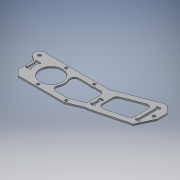
# Autodesk Inventor part: 足首_メインフレーム_1_1
Saved by Autodesk Inventor 2018 (Build 220112000, 112)
## iProperties
Created: 2016-04-30
Part Number: 足首_メインフレーム_1_1
Material: アルミニウム 2014-T4
Document SubType Name: Modeling
Designer: hiroaki
Density: 2.8 g/cm^3
Appearance: サテン
Mass: 6.61842 g
Surface Area: 42.008 cm^2
Volume: 2.36372 cm^3
d0: 1.000 ul
d1: 3.100 mm
d2: 3.000 mm
d3: 11.000 mm
d4: 0.025 mm
d5: 2.100 mm
d6: 21.500 mm
d7: 2.000 mm
d9: 10.000 mm
d11: 10.000 mm
d14: 0.025 mm
d15: 2.100 mm
d18: 22.000 mm
d20: 2.000 mm
d21: 0.025 mm
d22: 5.600 mm
d23: 1.000 mm
d25: 1.000 mm
d27: 5.000 mm
d28: 5.000 mm
d29: 2.000 mm
d30: 5.000 mm
d31: 5.000 mm
d32: 135.00 deg
d33: 1.500 mm
d34: 0.00 deg
d35: 6.100 mm
d36: 2.100 mm
d37: 6.000 ul
d39: 360.00 deg
d41: 0.250 mm
d42: 0.00 deg
d43: 3.500 mm
Author: hiroaki
Autodesk Inventor part; units mm, degrees
ref_plane "YZ Plane" through (0, 0, 0) normal (1, 0, 0) x (0, 1, 0)
ref_plane "XZ Plane" through (0, 0, 0) normal (0, 1, 0) x (-1, 0, 0)
ref_plane "XY Plane" through (0, 0, 0) normal (0, 0, 1) x (1, 0, 0)
derived "下半身全体像_1_1.ipt"
sketch "スケッチ1" plane through (0, 0, 0) normal (0, 0, 1) x (1, 0, 0)
  circle A0 centre (0, 0) radius 10.5 construction
  line L0 (0, 0) -> (-12, 0) construction
  arc A1 (0, 16) -> (-12, 10.583) centre (0, 0) ccw construction
  arc A2 (-12, -10.583) -> (0, -16) centre (0, 0) ccw construction
  line L1 (0, 16) -> (39.5, 16) construction
  line L2 (39.5, 16) -> (39.5, -16) construction
  line L3 (39.5, -16) -> (0, -16) construction
  circle A3 centre (1, 13.5) radius 1.35 projected
  circle A4 centre (1, -13.5) radius 1.35 projected
  circle A5 centre (28, 13.5) radius 1.35 projected
  circle A6 centre (28, -13.5) radius 1.35 projected
  line L4 (1, 13.5) -> (1, -13.5) construction
  line L5 (1, -13.5) -> (28, -13.5) construction
  line L6 (1, 13.5) -> (28, 13.5) construction
  line L7 (28, 13.5) -> (28, -13.5) construction
  line L8 (0, 0) -> (1, 0) construction
  line L9 (32, 120) -> (32, 20) construction
  line L10 (0, 0) -> (0, 0) construction
  circle A7 centre (32, 120) radius 4.05 projected
  line L11 (0, 140) -> (0, 40) construction
  circle A8 centre (0, 40) radius 4.05 projected
  line L12 (0, 0) -> (0, -100) construction
  line L13 (32, 20) -> (32, -80) construction
  line L14 (0, 0) -> (0, 40) construction
  circle A9 centre (32, 20) radius 6.5 construction
  line L15 (32, 23.5218) -> (35.05, 21.7609) construction
  line L16 (35.05, 21.7609) -> (35.05, 18.2391) construction
  line L17 (35.05, 18.2391) -> (32, 16.4782) construction
  line L18 (32, 16.4782) -> (28.95, 18.2391) construction
  line L19 (28.95, 18.2391) -> (28.95, 21.7609) construction
  line L20 (28.95, 21.7609) -> (32, 23.5218) construction
  line L21 (21.5, 152) -> (61, 152) construction
  line L22 (61, 152) -> (61, 100.5) construction
  line L23 (61, 100.5) -> (21.5, 100.5) construction
  line L24 (21.5, 100.5) -> (21.5, 152) construction
  line L25 (21.5, 140) -> (61, 140) construction
  line L26 (16, 150.5) -> (66.5, 150.5) construction
  line L27 (66.5, 150.5) -> (66.5, 129.5) construction
  line L28 (66.5, 129.5) -> (16, 129.5) construction
  line L29 (16, 129.5) -> (16, 150.5) construction
  circle A10 centre (0, 140) radius 10.5 construction
  line L30 (-13.5, 139) -> (13.5, 139) construction
  line L31 (13.5, 139) -> (13.5, 112) construction
  line L32 (13.5, 112) -> (-13.5, 112) construction
  line L33 (-13.5, 112) -> (-13.5, 139) construction
  circle A11 centre (-13.5, 139) radius 1.35 projected
  circle A12 centre (13.5, 139) radius 1.35 projected
  circle A13 centre (-13.5, 112) radius 1.35 projected
  circle A14 centre (13.5, 112) radius 1.35 projected
  line L34 (-12, 10.583) -> (-12, -10.583) construction
  circle A15 centre (0, -100) radius 4.05 construction
  circle A16 centre (32, -80) radius 4.05 construction
  circle A17 centre (0, -100) radius 10.5 construction
  line L35 (32, -80) -> (0, -100) construction
  line L36 (45, -60.5) -> (77.5, -60.5) construction
  line L37 (77.5, -60.5) -> (77.5, -112) construction
  line L38 (77.5, -112) -> (45, -112) construction
  line L39 (45, -112) -> (45, -60.5) construction
  line L40 (45, -100) -> (77.5, -100) construction
  line L41 (39.5, -89.5) -> (83, -89.5) construction
  line L42 (83, -89.5) -> (83, -110.5) construction
  line L43 (83, -110.5) -> (39.5, -110.5) construction
  line L44 (39.5, -110.5) -> (39.5, -89.5) construction
  line L45 (1, -86.5) -> (28, -86.5) construction
  line L46 (28, -86.5) -> (28, -113.5) construction
  line L47 (28, -113.5) -> (1, -113.5) construction
  line L48 (1, -113.5) -> (1, -86.5) construction
  circle A18 centre (1, -86.5) radius 1.35 projected
  circle A19 centre (1, -113.5) radius 1.35 projected
  circle A20 centre (28, -113.5) radius 1.35 projected
  circle A21 centre (28, -86.5) radius 1.35 projected
  circle A22 centre (32, 20) radius 4.05 projected
  circle A23 centre (32, 20) radius 4.05 projected
  line L49 (10.583, 152) -> (-10.583, 152) construction
  line L50 (16, 140) -> (16, 100.5) construction
  line L51 (16, 100.5) -> (-16, 100.5) construction
  line L52 (-16, 100.5) -> (-16, 140) construction
  arc A24 (16, 140) -> (10.583, 152) centre (0, 140) ccw construction
  arc A25 (-10.583, 152) -> (-16, 140) centre (0, 140) ccw construction
  line L53 (-12, -89.417) -> (-12, -110.583) construction
  line L54 (0, -84) -> (39.5, -84) construction
  line L55 (39.5, -84) -> (39.5, -116) construction
  line L56 (39.5, -116) -> (0, -116) construction
  arc A26 (0, -84) -> (-12, -89.417) centre (0, -100) ccw construction
  arc A27 (-12, -110.583) -> (0, -116) centre (0, -100) ccw construction
  circle A28 centre (-8.5, 0) radius 1.35 projected
  circle A29 centre (0, 0) radius 8.5 construction
  line L57 (35.05, 121.7609) -> (35.05, 118.2391) construction
  line L58 (35.05, 118.2391) -> (32, 116.4782) construction
  line L59 (32, 116.4782) -> (28.95, 118.2391) construction
  line L60 (28.95, 118.2391) -> (28.95, 121.7609) construction
  line L61 (28.95, 121.7609) -> (32, 123.5218) construction
  line L62 (32, 123.5218) -> (35.05, 121.7609) construction
  line L63 (0, 152) -> (0, 140) construction
  line L64 (0, 140) -> (0, 139) construction
  circle A30 centre (83.3, -84.5) radius 1.55
  line L65 (-19, -94.5) -> (-16, -94.5) construction
  line L66 (-16, -94.5) -> (-16, -105.5) construction
  line L67 (-16, -105.5) -> (-19, -105.5) construction
  line L68 (-19, -105.5) -> (-19, -94.5) construction
  line L69 (-15.975, -94.475) -> (-19.025, -94.475) construction
  line L70 (-19.025, -94.475) -> (-19.025, -105.525) construction
  line L71 (-19.025, -105.525) -> (-15.975, -105.525) construction
  line L72 (-15.975, -105.525) -> (-15.975, -94.475) construction
  circle A31 centre (-19.025, -95.525) radius 1.05 construction
  arc A32 (-19.025, -94.475) -> (-19.025, -96.575) centre (-19.025, -95.525) ccw
  line L73 (-19.025, -94.475) -> (-15.975, -94.475)
  arc A33 (-15.975, -96.575) -> (-15.975, -94.475) centre (-15.975, -95.525) ccw
  line L74 (-17.5, -94.475) -> (-17.5, -105.525) construction
  line L75 (-15.975, -96.575) -> (-15.975, -103.425)
  line L76 (-19.025, -96.575) -> (-19.025, -103.425)
  arc A34 (-19.025, -103.425) -> (-19.025, -105.525) centre (-19.025, -104.475) ccw
  arc A35 (-15.975, -105.525) -> (-15.975, -103.425) centre (-15.975, -104.475) ccw
  line L77 (-19.025, -105.525) -> (-15.975, -105.525)
  circle A36 centre (0, -100) radius 10.75
  line L78 (43, -95) -> (45, -95) construction
  line L79 (45, -95) -> (45, -105) construction
  line L80 (45, -105) -> (43, -105) construction
  line L81 (43, -105) -> (43, -95) construction
  line L82 (45, -95) -> (39.5, -95) construction
  line L83 (39.5, -95) -> (39.5, -105) construction
  line L84 (39.5, -105) -> (45, -105) construction
  line L85 (45, -105) -> (45, -95) construction
  line L86 (45.025, -94.975) -> (42.975, -94.975) construction
  line L87 (42.975, -94.975) -> (42.975, -105.025) construction
  line L88 (42.975, -105.025) -> (45.025, -105.025) construction
  line L89 (45.025, -105.025) -> (45.025, -94.975) construction
  circle A37 centre (42.975, -96.025) radius 1.05 construction
  line L90 (42.975, -94.975) -> (45.025, -94.975)
  arc A38 (42.975, -94.975) -> (42.975, -97.075) centre (42.975, -96.025) ccw
  arc A39 (45.025, -97.075) -> (45.025, -94.975) centre (45.025, -96.025) ccw
  line L91 (44, -95) -> (44, -105.025) construction
  line L92 (42.975, -97.075) -> (42.975, -102.925)
  line L93 (45.025, -97.075) -> (45.025, -102.925)
  line L94 (42.975, -105.025) -> (45.025, -105.025)
  arc A40 (42.975, -102.925) -> (42.975, -105.025) centre (42.975, -103.975) ccw
  arc A41 (45.025, -105.025) -> (45.025, -102.925) centre (45.025, -103.975) ccw
  line L95 (77.5, -96.5) -> (45, -96.5) construction
  line L96 (77.5, -74.5) -> (79.5, -74.5) construction
  line L97 (79.5, -74.5) -> (79.5, -96.5) construction
  line L98 (79.5, -96.5) -> (77.5, -96.5) construction
  line L99 (77.5, -96.5) -> (77.5, -74.5) construction
  line L100 (45, -74.5) -> (77.5, -74.5) construction
  line L101 (79.525, -74.475) -> (77.475, -74.475) construction
  line L102 (77.475, -74.475) -> (77.475, -96.525) construction
  line L103 (77.475, -96.525) -> (79.525, -96.525) construction
  line L104 (79.525, -96.525) -> (79.525, -74.475) construction
  circle A42 centre (77.475, -75.525) radius 1.05 construction
  line L105 (77.475, -74.475) -> (79.525, -74.475)
  arc A43 (77.475, -74.475) -> (77.475, -76.575) centre (77.475, -75.525) ccw
  line L106 (77.475, -76.575) -> (77.475, -94.425)
  arc A44 (79.525, -76.575) -> (79.525, -74.475) centre (79.525, -75.525) ccw
  line L107 (79.525, -76.575) -> (79.525, -94.425)
  line L108 (78.5, -74.475) -> (78.5, -89.5) construction
  line L109 (79.525, -85.5) -> (77.475, -85.5) construction
  arc A45 (77.475, -94.425) -> (77.475, -96.525) centre (77.475, -95.475) ccw
  line L110 (77.475, -96.525) -> (79.525, -96.525)
  arc A46 (79.525, -96.525) -> (79.525, -94.425) centre (79.525, -95.475) ccw
  line L111 (83.3, -81.2668) -> (86.1, -82.8834) construction
  line L112 (86.1, -82.8834) -> (86.1, -86.1166) construction
  line L113 (86.1, -86.1166) -> (83.3, -87.7332) construction
  line L114 (83.3, -87.7332) -> (80.5, -86.1166) construction
  line L115 (80.5, -86.1166) -> (80.5, -82.8834) construction
  line L116 (80.5, -82.8834) -> (83.3, -81.2668) construction
  line L117 (-21, -95.2931) -> (-21, -110.5)
  line L118 (-21, -110.5) -> (-16, -116)
  line L119 (-16, -116) -> (28.4967, -116)
  line L120 (28.4967, -116) -> (43, -110)
  line L121 (43, -110) -> (45, -110)
  line L122 (87.1, -85.3494) -> (87.1, -75.6858)
  line L123 (76.7437, -69.5) -> (39.5, -84)
  line L124 (39.5, -84) -> (-16, -84)
  circle A47 centre (1, -86.5) radius 2.5 construction
  circle A48 centre (28, -113.5) radius 2.5 construction
  circle A49 centre (43, -110) radius 2 construction
  circle A50 centre (79.5, -101.5) radius 1 construction
  line L125 (80.9142, -69.5) -> (87.1, -75.6858)
  circle A51 centre (79.5, -69.5) radius 1 construction
  line L126 (76.7437, -69.5) -> (80.9142, -69.5)
  line L127 (45, -110) -> (77.5, -101.5)
  line L128 (77.5, -101.5) -> (79.5, -101.5)
  line L129 (79.5, -101.5) -> (87.1, -85.3494)
  circle A52 centre (83.3, -84.5) radius 3.8 construction
  line L130 (0, -100) -> (1, -100) construction
  line L131 (-19.5, -90.6166) -> (-22.3, -92.2332)
  line L132 (-22.3, -92.2332) -> (-25.1, -90.6166)
  line L133 (-25.1, -90.6166) -> (-25.1, -87.3834)
  line L134 (-25.1, -87.3834) -> (-22.3, -85.7668)
  line L135 (-22.3, -85.7668) -> (-19.5, -87.3834)
  line L136 (-19.5, -87.3834) -> (-19.5, -90.6166)
  circle A53 centre (-22.3, -89) radius 1.55
  line L137 (-21, -95.2931) -> (-27.1, -91.7713)
  line L138 (-27.1, -91.7713) -> (-27.1, -86.2287)
  line L139 (-27.1, -86.2287) -> (-23.2397, -84)
  line L140 (-23.2397, -84) -> (-16, -84)
  point P0 (66.5, 140)
  point P1 (39.5, 0)
  point P2 (83, -100)
  point P3 (-12, -100)
  point P4 (39.5, -100)
  point P5 (-19, -100)
  point P6 (39.5, -100)
  point P7 (78.5, -85.5)
  point P8 (-19.025, -100)
  dimension "d5" = 2.1
  dimension "d15" = 2.1
  dimension "d1" = 3.1
  dimension "d2" = 3
  dimension "d3" = 11
  dimension "d4" = 0.025
  dimension "d6" = 21.5
  dimension "d7" = 2
  dimension "d9" = 10
  dimension "d11" = 10
  dimension "d14" = 0.025
  dimension "d18" = 22
  dimension "d20" = 2
  dimension "d21" = 0.025
  dimension "d22" = 5.6
  dimension "d23" = 1
  dimension "d25" = 1
  dimension "d28" = 5
  dimension "d29" = 2
  dimension "d30" = 5
  dimension "d31" = 5
  dimension "d32" = 135
  dimension "d43" = 3.5
  dimension "d58" = 2
  dimension "d59" = 5
  dimension "d60" = 5.6
  dimension "d61" = 3.1
  dimension "d64" = 0.5
  dimension "d65" = 2
  dimension "d66" = 2
  dimension "d67" = 5.5
  dimension "d68" = 2
  dimension "d76" = 1
  dimension "d77" = 4
  constraints: 152 end point, 24 point on circle, 21 centre point, 18 parallel, 15 horizontal, 15 point on line, 14 perpendicular, 13 collinear, 12 midpoint, 11 tangent, 10 vertical, 10 vertical alignment, 9 coincident, 9 symmetric about line, 7 equal radius, 2 horizontal alignment, 53 other
  measures "d1" diameter of A30
  measures "d2" distance of L65.start L65.end
  measures "d3" distance of L67.end L65.start
  measures "d4" distance between parallel lines of L69 L65
  measures "d6" diameter of A36
  measures "d7" distance of L78.start L78.end
  measures "d9" distance of L82.end L83.end
  measures "d11" distance of L80.end L78.start
  measures "d14" distance between parallel lines of L86 L78
  measures "d18" distance between parallel lines of L100 L95
  measures "d20" distance of L96.start L96.end
  measures "d21" distance between parallel lines of L101 L96
  measures "d22" distance between parallel lines of L115 L112
  measures "d23" distance between parallel lines of L115 L97
  measures "d25" distance between parallel lines of L122 L112
  measures "d28" distance of L80.end A49.centre
  measures "d29" diameter of A50
  measures "d30" distance of L97.end A50.centre
  measures "d31" distance of L96.end A51.centre
  measures "d32" angle of L122 L125
  measures "d43" distance between parallel lines of L95 L40
  measures "d58" distance between parallel lines of L68 L117
  measures "d59" distance from line of L117.end L67
  measures "d60" distance between parallel lines of L135 L132
  measures "d61" diameter of A53
  measures "d64" distance between parallel lines of L136 L68
  measures "d65" distance between parallel lines of L137 L132
  measures "d66" distance between parallel lines of L133 L138
  measures "d67" distance from line of L65 point (-22.3, -89)
  measures "d68" distance between parallel lines of L134 L139
  measures "d76" distance from line of L109 A30.centre
  measures "d77" distance between parallel lines of L53 L66
extrude "押し出し1" add sketch "スケッチ1" along normal blind 1.5 contours L137 L138 L139 L140 L124 L123 L126 L125 L122 L129 L128 L127 L121 L120 L119 L118 L117 | L131 L132 L133 L134 L135 L136
sketch "スケッチ3" plane through (39.5, -84, 0) normal (0, 0, -1) x (-1, 0, 0)
  circle A0 centre (-43.8, -0.5) radius 1.55 projected
  line L0 (-40.75, 1.2609) -> (-40.75, -2.2609)
  line L1 (-40.75, -2.2609) -> (-43.8, -4.0218)
  line L2 (-43.8, -4.0218) -> (-46.85, -2.2609)
  line L3 (-46.85, -2.2609) -> (-46.85, 1.2609)
  line L4 (-46.85, 1.2609) -> (-43.8, 3.0218)
  line L5 (-43.8, 3.0218) -> (-40.75, 1.2609)
  circle A1 centre (-43.8, 1.9718) radius 1.05
  circle A2 centre (-45.9407, 0.7359) radius 1.05
  circle A3 centre (-45.9407, -1.7359) radius 1.05
  circle A4 centre (-43.8, -2.9718) radius 1.05
  circle A5 centre (-41.6593, -1.7359) radius 1.05
  circle A6 centre (-41.6593, 0.7359) radius 1.05
  circle A7 centre (61.8, -5) radius 1.55 projected
  line L6 (64.6, -6.6166) -> (61.8, -8.2332)
  line L7 (61.8, -8.2332) -> (59, -6.6166)
  line L8 (59, -6.6166) -> (59, -3.3834)
  line L9 (59, -3.3834) -> (61.8, -1.7668)
  line L10 (61.8, -1.7668) -> (64.6, -3.3834)
  line L11 (64.6, -3.3834) -> (64.6, -6.6166)
  circle A8 centre (61.8, -2.8168) radius 1.05
  circle A9 centre (59.9093, -3.9084) radius 1.05
  circle A10 centre (59.9093, -6.0916) radius 1.05
  circle A11 centre (61.8, -7.1832) radius 1.05
  circle A12 centre (63.6907, -6.0916) radius 1.05
  circle A13 centre (63.6907, -3.9084) radius 1.05
  point P0 (39.5, 84)
  point P1 (-43.8, -0.5)
  point P2 (-46.85, 1.2609)
  point P3 (-46.85, -2.2609)
  point P4 (-43.8, -4.0218)
  point P5 (-40.75, -2.2609)
  point P6 (-40.75, 1.2609)
  point P7 (59, -3.3834)
  point P8 (59, -6.6166)
  point P9 (61.8, -8.2332)
  point P10 (64.6, -6.6166)
  point P11 (64.6, -3.3834)
  dimension "d36" = 2.1
  dimension "d69" = 2.1
  dimension "d35" = 6.1
  dimension "d39" = 360
  dimension "d72" = 360
  dimension "d74" = 5.6
  constraints: 24 end point, 6 vertical alignment, 2 coincident, 2 vertical, 96 other
  measures "d35" distance between parallel lines of L3 L0
  measures "d74" distance between parallel lines of L11 L8
extrude "押し出し2" cut sketch "スケッチ3" against normal blind 0.25 contours A0 A6 L0 A5 | A6 A0 | A0 A6 L5 L0 | A5 L0 L1 A0 | A0 A5 | A0 A1 L5 A6 | L0 A6 | A5 L1 A4 A0 | A5 L0 | A1 A0 | A0 A1 L4 L5 | A6 L5 | A4 L1 L2 A0 | A0 A4 | L1 A5 | A0 A2 L4 A1 | L5 A1 | A4 L2 A3 A0 | A4 L1 | A2 A0 | A0 A2 L3 L4 | A1 L4 | A3 L2 L3 A0 | A0 A3 | L2 A4 | A0 A3 L3 A2 | L4 A2 | A3 L2 | A2 L3 | L3 A3 | A7 A13 L11 A12 | A13 A7 | A7 A13 L10 L11 | A12 L11 L6 A7 | A7 A12 | A7 A8 L10 A13 | L11 A13 | A12 L6 A11 A7 | A12 L11 | A8 A7 | A7 A8 L9 L10 | A13 L10 | A11 L6 L7 A7 | A7 A11 | L6 A12 | A7 A9 L9 A8 | L10 A8 | A11 L7 A10 A7 | A11 L6 | A9 A7 | A7 A9 L8 L9 | A8 L9 | A10 L7 L8 A7 | A7 A10 | L7 A11 | A7 A10 L8 A9 | L9 A9 | A10 L7 | A9 L8 | L8 A10
sketch "スケッチ4" plane through (-23.2397, -84, 1.5) normal (0, 0, 1) x (1, 0, 0)
  circle A0 centre (23.2397, -16) radius 10.75 projected
  line L0 (102.7647, -12.525) -> (100.7147, -12.525) projected
  line L1 (100.7147, 9.525) -> (102.7647, 9.525) projected
  line L2 (68.2647, -21.025) -> (66.2147, -21.025) projected
  line L3 (66.2147, -18.925) -> (66.2147, -13.075) projected
  line L4 (66.2147, -10.975) -> (68.2647, -10.975) projected
  circle A1 centre (51.2397, -2.5) radius 1.35 projected
  circle A2 centre (51.2397, -29.5) radius 1.35 projected
  line L5 (62.7397, 0) -> (0, 0) projected
  line L6 (51.7365, -32) -> (66.2397, -26) projected
  line L7 (68.2397, -26) -> (100.7397, -17.5) projected
  line L8 (99.9834, 14.5) -> (62.7397, 0) projected
  line L9 (29.6866, -5) -> (49.5814, -5)
  arc A3 (49.5814, -5) -> (52.8981, -5) centre (51.2397, -2.5) ccw
  arc A4 (29.6866, -27) -> (29.6866, -5) centre (23.2397, -16) ccw
  line L10 (52.8981, -5) -> (63.2397, -5)
  line L11 (63.2397, -5) -> (63.2397, -21.8301)
  line L12 (63.2397, -21.8301) -> (51.8164, -26.5559)
  arc A5 (51.8164, -26.5559) -> (49.5814, -27) centre (51.2397, -29.5) ccw
  line L13 (29.6866, -27) -> (29.6866, -27)
  line L14 (29.6866, -27) -> (49.5814, -27)
  line L15 (23.2397, -16) -> (66.2147, -16) construction
  line L16 (67.2397, -10.975) -> (67.2397, -21.025) construction
  line L17 (71.2397, -2.0563) -> (71.2397, -20.0472)
  line L18 (71.2397, -20.0472) -> (97.7397, -13.1164)
  line L19 (97.7397, -13.1164) -> (97.7397, 8.2609)
  line L20 (97.7397, 8.2609) -> (71.2397, -2.0563)
  line L21 (101.7397, 9.525) -> (101.7397, -12.525) construction
  point P0 (23.2397, 84)
  dimension "d44" = 5
  dimension "d46" = 2
  dimension "d48" = 3
  dimension "d49" = 4
  dimension "d50" = 5
  dimension "d51" = 4
  dimension "d52" = 4
  dimension "d53" = 5
  dimension "d54" = 5
  constraints: 26 end point, 6 point on circle, 5 midpoint, 4 parallel, 3 centre point, 3 coincident, 2 horizontal, 2 perpendicular, 2 vertical, 1 equal radius, 1 horizontal alignment, 1 symmetric about line, 1 vertical alignment
  measures "d44" distance between parallel lines of L5 L9
  measures "d46" radial gap between concentric circles of A4 A0
  measures "d48" radius of A3
  measures "d49" distance between parallel lines of L16 L11
  measures "d50" distance between parallel lines of L6 L12
  measures "d51" distance between parallel lines of L16 L17
  measures "d52" distance between parallel lines of L21 L19
  measures "d53" distance between parallel lines of L8 L20
  measures "d54" distance between parallel lines of L7 L18
extrude "押し出し3" cut sketch "スケッチ4" against normal blind 10 contours L9 A3 L10 L11 L12 A5 L14 A4 | L20 L19 L18 L17
fillet "フィレット1" radius 4 12 edges at (40, -89, 0.75) (29.6583, -89, 0.75) (26.3417, -89, 0.75) (26.3417, -111, 0.75) (28.5767, -110.5559, 0.75) (40, -105.8301, 0.75) (48, -104.0472, 0.75) (48, -86.0563, 0.75) (74.5, -75.7391, 0.75) (74.5, -97.1164, 0.75) (6.4469, -111, 0.75) (6.4469, -89, 0.75)
fillet "フィレット2" radius 2 7 edges at (-21, -95.2931, 0.75) (-27.1, -91.7713, 0.75) (-27.1, -86.2287, 0.75) (-23.2397, -84, 0.75) (-21, -110.5, 0.75) (-16, -116, 0.75) (39.5, -84, 0.75)
equation "\"d20\" = d7"
equation "\"d31\" = d30"
